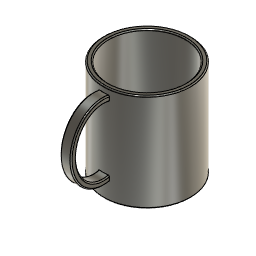
kaffe kopp (Autodesk Fusion 360 design; units mm, degrees)
Autodesk Fusion 360 part; units mm, degrees
cylinder "CylinderPrimitive1" add diameter 80 height 90 placed x (1, 0, 0) y (0, 1, 0) z (0, 0, 1) at (60, 60, 0)
ref_plane "WorkPlane1" through (55, 0, 0) normal (1, 0, 0) x (0, 1, 0)
sketch "Sketch2" plane through (55, 0, 0) normal (1, 0, 0) x (0, 1, 0)
  ellipse E0 centre (15, 50) end of major axis (15, 15) minor radius 30
  line L0 (15, 85) -> (15, 15)
  line L1 (-15, 50) -> (45, 50)
  ellipse E1 centre (15, 50) end of major axis (15, 20) minor radius 25
  line L2 (15, 80) -> (15, 20)
  line L3 (-10, 50) -> (40, 50)
  constraint vertical L0
  constraint coincident E0 L0.start
  constraint coincident E0 L0.end
  constraint coincident E0 L1.start
  constraint coincident E0 L1.end
  constraint concentric E0 E1
  constraint perpendicular L1 L2
  constraint coincident E1 L2.start
  constraint coincident E1 L2.end
  constraint coincident E1 L3.start
  constraint coincident E1 L3.end
extrude "Extrude1" add sketch "Sketch2" along normal blind 10 contours E0 L0 L1 E1 | E0 L0 L1 E1 | E0 L0 L1 E1 | E0 L0 L1 E1
sketch "Sketch3" plane through (0, 0, 90) normal (0, 0, 1) x (-1, 0, 0)
  circle A0 centre (-60, -60) radius 40
  circle A1 centre (-60, -60) radius 35.3553
  constraint concentric A0 A1
extrude "Extrude2" cut sketch "Sketch3" against normal blind 85 contours A1
fillet "Fillet1" radius 1 6 edges at (92.9627, 47.215, 90) (22.7069, 45.5354, 90) (65, -10, 50) (55, -10, 50) (55, -15, 50) (65, -15, 50)
fillet "Fillet2" radius 1 1 edges at (22.7069, 74.4646, 0)
